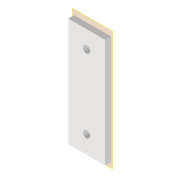
# Autodesk Inventor part: 40_microfluidic_chip_lightsheet_layer1_negative_mould_lower_v0
Saved by Autodesk Inventor 2022 (Build 260153000, 153)
## iProperties
Created: 2021-12-21
Part Number: 40_microfluidic_chip_lightsheet_layer1_negative_mould_lower_v0
Material: Generisch
Document SubType Name: Modeling
Designer: diederichbenedict
Density: 1 g/cm^3
Appearance: Vorgabe
Author: diederichbenedict
Autodesk Inventor part; units mm, degrees
ref_plane "YZ Plane" through (0, 0, 0) normal (1, 0, 0) x (0, 1, 0)
ref_plane "XZ Plane" through (0, 0, 0) normal (0, 1, 0) x (-1, 0, 0)
ref_plane "XY Plane" through (0, 0, 0) normal (0, 0, 1) x (1, 0, 0)
ref_plane "Arbeitsebene1" through (0, 0, 0) normal (0, 0, 1) x (1, 0, 0)
sketch "Skizze1" plane through (0, 0, 0) normal (0, 0, 1) x (1, 0, 0)
  circle A0 centre (0, -25) radius 2.5 projected
  circle A1 centre (0, 25) radius 2.5 projected
  line L0 (12.5, -37) -> (12.5, 37) projected
  line L1 (12.5, 37) -> (-12.5, 37) projected
  line L2 (-12.5, 37) -> (-12.5, -37) projected
  line L3 (-12.5, -37) -> (12.5, -37) projected
  line L4 (0.75, -9.25) -> (-0.75, -9.25) projected
  line L5 (-0.75, -9.25) -> (-0.75, 9.25) projected
  line L6 (-0.75, 9.25) -> (0.75, 9.25) projected
  line L7 (0.75, 9.25) -> (0.75, -9.25) projected
  circle A2 centre (8.5, -30) radius 1.4 projected
  circle A3 centre (-8.5, -30) radius 1.4 projected
  circle A4 centre (-8.5, 30) radius 1.4 projected
  circle A5 centre (8.5, 30) radius 1.4 projected
  point P0 (0, 0)
extrude "Extrusion1" add sketch "Skizze1" along normal blind 4 contours L3 L2 L1 L0 | L4 L5 L6 L7 | A2 | A3 | A4 | A5
sketch "Skizze2" plane through (0, 0, 0) normal (0, 0, -1) x (-1, 0, 0)
  line L0 (9.25, 9.25) -> (-9.25, 9.25) projected
  line L1 (9.25, -9.25) -> (9.25, 9.25) projected
  line L2 (-9.25, -9.25) -> (9.25, -9.25) projected
  line L3 (-9.25, 9.25) -> (-9.25, -9.25) projected
  point P0 (0, 0)
extrude "Extrusion2" add sketch "Skizze2" along normal blind 0.3
sketch "Skizze3" plane through (0, 0, -0.3) normal (0, 0, -1) x (-1, 0, 0)
  line L0 (0.75, 7.25) -> (-0.75, 7.25) projected
  line L1 (0.75, -23.701) -> (0.75, 23.701) projected
  line L2 (-0.75, 23.701) -> (-0.75, -23.701) projected
  line L3 (-0.75, -7.25) -> (0.75, -7.25) projected
  line L4 (0.75, 7.25) -> (-0.75, 7.25)
  line L5 (-0.75, 7.25) -> (-0.75, -7.25)
  line L6 (-0.75, -7.25) -> (0.75, -7.25)
  line L7 (0.75, -7.25) -> (0.75, 7.25)
  point P0 (0, 0)
  constraints: 8 end point, 2 parallel, 1 horizontal, 1 perpendicular
extrude "Extrusion3" add sketch "Skizze3" along normal blind 0.3
